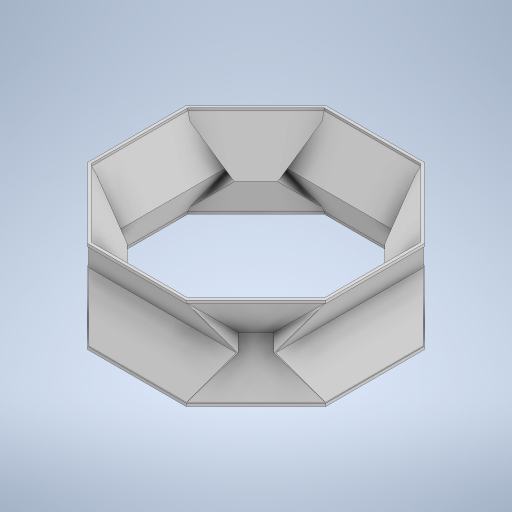
# Autodesk Inventor part: 팔각형 OV-PAM 층 한개
Saved by Autodesk Inventor 2024 (Build 280153000, 153)
## iProperties
Created: 2023-06-16
Part Number: 팔각형 OV-PAM 층 한개
Material: 일반
Document SubType Name: Modeling
Designer: jsw
Density: 1 g/cm^3
Appearance: 기본값
Author: jsw
Autodesk Inventor part; units mm, degrees
ref_plane "YZ Plane" through (0, 0, 0) normal (1, 0, 0) x (0, 1, 0)
ref_plane "XZ Plane" through (0, 0, 0) normal (0, 1, 0) x (-1, 0, 0)
ref_plane "XY Plane" through (0, 0, 0) normal (0, 0, 1) x (1, 0, 0)
sketch "스케치1" plane through (0, 0, 0) normal (0, 1, 0) x (-1, 0, 0)
  line L0 (-32.5919, 13.5) -> (-13.5, 32.5919)
  line L1 (-13.5, 32.5919) -> (13.5, 32.5919)
  line L2 (13.5, 32.5919) -> (32.5919, 13.5)
  line L3 (32.5919, 13.5) -> (32.5919, -13.5)
  line L4 (32.5919, -13.5) -> (13.5, -32.5919)
  line L5 (13.5, -32.5919) -> (-13.5, -32.5919)
  line L6 (-13.5, -32.5919) -> (-32.5919, -13.5)
  line L7 (-32.5919, -13.5) -> (-32.5919, 13.5)
  line L8 (-13.6657, 32.9919) -> (13.6657, 32.9919)
  line L9 (13.6657, 32.9919) -> (32.9919, 13.6657)
  line L10 (32.9919, 13.6657) -> (32.9919, -13.6657)
  line L11 (32.9919, -13.6657) -> (13.6657, -32.9919)
  line L12 (13.6657, -32.9919) -> (-13.6657, -32.9919)
  line L13 (-13.6657, -32.9919) -> (-32.9919, -13.6657)
  line L14 (-32.9919, -13.6657) -> (-32.9919, 13.6657)
  line L15 (-32.9919, 13.6657) -> (-13.6657, 32.9919)
  point P0 (0, 0)
  point P1 (0, 0)
  point P2 (0, 0)
  dimension "d0" = 27
  dimension "d2" = 0.4
  constraints: 32 end point, 2 coincident, 2 horizontal, 34 other
  measures "d0" distance of L0.end L1.end
  measures "d2" distance between parallel lines of L10 L3
extrude "돌출2" add sketch "스케치1" along normal blind 12 contours L0 L1 L2 L3 L4 L5 L6 L7 | L8 L9 L10 L11 L12 L13 L14 L15
ref_plane "작업 평면2" through (32.9919, 0, 13.6657) normal (-0.8660254, -0.5, 0) x (0, 0, -1)
sketch "스케치3" plane through (32.9919, 0, 13.6657) normal (1, 0, 0) x (0, 0, -1)
  line L0 (0, 0) -> (0, 12) projected
  line L1 (0, 12) -> (27.3314, 12) projected
  line L2 (0, 0) -> (27.3314, 0)
  line L3 (27.3314, 0) -> (27.3314, 12)
  line L4 (27.3314, 12) -> (0, 12)
  line L5 (0, 12) -> (0, 0)
  line L6 (0, 12) -> (-7.3047, 12)
  line L7 (-19.3262, 12) -> (0, 12) projected
  line L8 (0, 0) -> (-7.3047, 12)
  line L9 (27.3314, 12) -> (34.6361, 12)
  line L10 (34.6361, 12) -> (27.3314, 0)
  point P0 (13.6657, 0)
  dimension "d17" = 121.33
  dimension "d18" = 121.33
  constraints: 16 end point, 2 parallel, 2 point on line, 1 horizontal, 1 perpendicular
  measures "d17" angle of L8 L2
  measures "d18" angle of L2 L10
extrude "돌출4" cut sketch "스케치3" against normal up to surface surface through (32.9919, 0, 13.6657) normal (-0.8660254, -0.5, 0)
sketch "스케치4" plane through (13.6657, 0, 32.9919) normal (0.7071068, 0, 0.7071068) x (0.7071068, 0, -0.7071068)
  line L0 (0, 0) -> (0, 12) projected
  line L1 (27.3314, 0) -> (27.3314, 12) projected
  line L2 (0, 0) -> (27.3314, 0)
  line L3 (27.3314, 0) -> (27.3314, 12)
  line L4 (27.3314, 12) -> (0, 12)
  line L5 (0, 12) -> (0, 0)
  line L6 (27.3314, 0) -> (17.5334, 12) projected
  line L7 (27.3314, 0) -> (17.1657, 12)
  line L8 (27.3314, 0) -> (0, 0) projected
  line L9 (0, 0) -> (10.1657, 12)
  line L10 (27.3314, 12) -> (0, 12) projected
  point P0 (13.6657, 0)
  point P1 (13.6657, 12)
  dimension "d40" = 7
  dimension "d41" = 3.5
  constraints: 12 end point, 2 parallel, 2 point on line, 1 horizontal, 1 midpoint, 1 perpendicular
  measures "d40" distance of L9.end L7.end
  measures "d41" distance of L7.end point (13.666, 12)
ref_plane "작업 평면3" through (13.6657, 0, 32.9919) normal (0.6123724, 0.5, 0.6123724) x (0.7071068, 0, -0.7071068)
extrude "돌출5" cut sketch "스케치4" against normal up to surface contours L9 L4 L7 L2 surface through (13.6657, 0, 32.9919) normal (0.6123724, 0.5, 0.6123724)
pattern_circular "원형 패턴1" count 4 over 360 about axis through (0, -10, 0) along (0, 1, 0) of "돌출4"
pattern_circular "원형 패턴2" count 4 over 360 about axis through (0, -10, 0) along (0, 1, 0) of "돌출5"
mirror "미러5" about plane through (0, 12, 0) normal (0, 1, 0) of "돌출2", "돌출5", "원형 패턴2", "돌출4", "원형 패턴1"
ref_plane "작업 평면5" through (-13.6657, 12, -32.9919) normal (0, 1, 0) x (1, 0, 0)
sketch "스케치9" plane through (-13.6657, 24, -32.9919) normal (0, 1, 0) x (1, 0, 0)
  line L0 (46.6576, -46.6576) -> (46.6576, -19.3262) projected
  line L1 (46.6576, -19.3262) -> (27.3314, 0) projected
  line L2 (27.3314, 0) -> (0, 0) projected
  line L3 (0, 0) -> (-19.3262, -19.3262) projected
  line L4 (-19.3262, -19.3262) -> (-19.3262, -46.6576) projected
  line L5 (-19.3262, -46.6576) -> (0, -65.9838) projected
  line L6 (0, -65.9838) -> (27.3314, -65.9838) projected
  line L7 (27.3314, -65.9838) -> (46.6576, -46.6576) projected
  point P0 (13.6657, -32.9919)
extrude "돌출8" add sketch "스케치9" along normal blind 0.8
mirror "미러7" about plane through (-13.6657, 12, -32.9919) normal (0, 1, 0) of "돌출8"
shell "쉘5" thickness 0.6 removed faces 2 at (-4.5552, 24.8, -10.9973) at (-4.5552, -0.8, -10.9973)
sketch "스케치10" plane through (-13.6657, -0.8, 32.9919) normal (0, -1, 0) x (1, 0, 0)
  line L0 (-0.0828, 0.2) -> (27.4142, 0.2)
  line L1 (27.4142, 0.2) -> (46.8576, -19.2434)
  line L2 (46.8576, -19.2434) -> (46.8576, -46.7404)
  line L3 (46.8576, -46.7404) -> (27.4142, -66.1838)
  line L4 (27.4142, -66.1838) -> (-0.0828, -66.1838)
  line L5 (-0.0828, -66.1838) -> (-19.5262, -46.7404)
  line L6 (-19.5262, -46.7404) -> (-19.5262, -19.2434)
  line L7 (-19.5262, -19.2434) -> (-0.0828, 0.2)
  line L8 (46.6576, -19.3262) -> (46.6576, -46.6576) projected
  line L9 (46.0576, -19.5747) -> (46.0576, -46.409) projected
  line L10 (46.0576, -46.409) -> (27.0828, -65.3838) projected
  line L11 (27.0828, -65.3838) -> (0.2485, -65.3838) projected
  line L12 (0.2485, -65.3838) -> (-18.7262, -46.409) projected
  line L13 (-18.7262, -46.409) -> (-18.7262, -19.5747) projected
  line L14 (-18.7262, -19.5747) -> (0.2485, -0.6) projected
  line L15 (0.2485, -0.6) -> (27.0828, -0.6) projected
  line L16 (27.0828, -0.6) -> (46.0576, -19.5747) projected
  line L17 (46.6576, -46.6576) -> (27.3314, -65.9838) projected
  line L18 (46.6576, -19.3262) -> (46.6576, -46.6576) projected
  line L19 (27.3314, 0) -> (46.6576, -19.3262) projected
  line L20 (0, 0) -> (27.3314, 0) projected
  line L21 (-19.3262, -19.3262) -> (0, 0) projected
  line L22 (-19.3262, -46.6576) -> (-19.3262, -19.3262) projected
  line L23 (0, -65.9838) -> (-19.3262, -46.6576) projected
  line L24 (27.3314, -65.9838) -> (0, -65.9838) projected
  point P0 (13.6657, -32.9919)
  point P1 (13.6657, -32.9919)
  dimension "d42" = 0.2
  constraints: 16 end point, 1 coincident, 1 horizontal, 17 other
  measures "d42" distance between parallel lines of L8 L2
extrude "돌출9" add sketch "스케치10" against normal blind 0.8 contours L0 L1 L2 L3 L4 L5 L6 L7
mirror "미러8" about plane through (-13.6657, 12, -32.9919) normal (0, 1, 0) of "돌출9"
equation "\"d41\" = 0.5 * d40"
